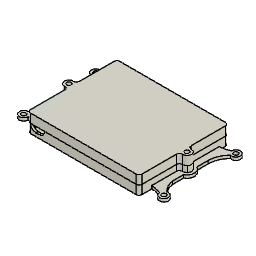
bat case v9 (Autodesk Fusion 360 design; units mm, degrees)
Autodesk Fusion 360 part; units mm, degrees
note: some values were not read from the file. Chosen so that the rebuilt part matches the saved one: which bodies a step acts on; which face or edge a step refers to; which pieces of a blend or face edit are solid. Set by a fixed rule: which sketch regions a step uses.
sketch "Sketch1" plane through (0, 0, 0) normal (0, 0, 1) x (1, 0, 0)
  line L0 (0, 0) -> (93.2, 0) construction
  line L1 (93.2, 0) -> (93.2, -48.6) construction
  line L2 (93.2, -48.6) -> (0, -48.6) construction
  line L3 (0, -48.6) -> (0, 0) construction
  line L4 (0, 0) -> (93.2, 0) construction
  line L5 (93.2, 0) -> (93.2, -48.6) construction
  line L6 (93.2, -48.6) -> (0, -48.6) construction
  line L7 (0, -48.6) -> (0, 0) construction
  line L8 (0, 0) -> (93.2, -48.6) construction
  line L9 (0, -48.6) -> (93.2, 0) construction
  line L10 (80.4585, 3.2151) -> (12.6326, -51.9036) construction
  line L11 (13.0397, 2.0949) -> (81.6326, -51.8528) construction
  circle A0 centre (93.2, 0) radius 1.5
  circle A1 centre (93.2, -48.6) radius 1.5
  circle A2 centre (0, -48.6) radius 1.5
  circle A3 centre (0, 0) radius 1.5
  circle A4 centre (0, 0) radius 3
  circle A5 centre (0, -48.6) radius 3
  circle A6 centre (93.2, -48.6) radius 3
  circle A7 centre (93.2, 0) radius 3
  line L12 (1.5, -2.5981) -> (1.5, -2.5138)
  line L13 (83.45, -54.15) -> (83.45, 3.05)
  line L14 (83.45, 3.05) -> (11.25, 3.05)
  line L15 (11.25, 3.05) -> (11.25, -54.15)
  line L16 (11.25, -54.15) -> (83.45, -54.15)
  line L17 (89.3079, -13.4947) -> (89.3079, -34.9816)
  line L18 (5.2688, -37.4913) -> (5.2688, -13.498)
  line L19 (9.7699, -1.523) -> (11.25, -1.523)
  line L20 (83.45, -1.523) -> (83.449, -1.523)
  line L21 (88.614, -49.274) -> (83.45, -49.274)
  line L22 (11.25, -47.288) -> (9.4012, -47.2941)
  arc A8 (9.4012, -47.2941) -> (2.9961, -48.7539) centre (9.4508, -62.2941) ccw
  arc A9 (5.2688, -13.498) -> (0.8586, -2.8745) centre (-9.7312, -13.498) ccw
  arc A10 (2.9986, 0.0924) -> (9.7699, -1.523) centre (9.7699, 13.477) ccw
  arc A11 (83.449, -1.523) -> (90.2011, 0.0827) centre (83.449, 13.477) ccw
  arc A12 (89.3079, -34.9816) -> (93.7677, -45.6542) centre (104.3079, -34.9816) ccw
  arc A13 (90.3003, -49.3691) -> (88.614, -49.274) centre (88.614, -64.274) ccw
  arc A14 (0.8858, -45.7338) -> (5.2688, -37.4913) centre (-8.9578, -35.2127) ccw
  arc A15 (92.3454, -2.8757) -> (89.3079, -13.4947) centre (104.6143, -12.1291) ccw
  line L23 (9.65, 4.65) -> (9.65, -55.75)
  line L24 (9.65, -55.75) -> (85.05, -55.75)
  line L25 (85.05, -55.75) -> (85.05, 4.65)
  line L26 (85.05, 4.65) -> (9.65, 4.65)
  point P0 (46.6, -24.3)
  dimension "d1" = 93.2
  dimension "d2" = 48.6
  dimension "d3" = 69
  dimension "d4" = 54
  dimension "d5" = 3
  dimension "d6" = 3
  dimension "d7" = 3
  dimension "d8" = 3
  dimension "d9" = 6
  dimension "d10" = 6
  dimension "d11" = 6
  dimension "d12" = 6
  dimension "d19" = 15
  dimension "d20" = 15
  dimension "d21" = 15
  dimension "d22" = 15
  dimension "d24" = 15
  dimension "d25" = 15
  dimension "d33" = 1.6
  constraint coincident L0.start L3.end
  constraint horizontal L0
  constraint perpendicular L0 L1
  constraint perpendicular L1 L2
  constraint perpendicular L0 L3
  constraint horizontal L4
  constraint vertical L5
  constraint horizontal L6
  constraint vertical L7
  constraint coincident L10 P0
  constraint coincident L11 P0
  constraint midpoint L9 P0
  constraint coincident L0.end L1.start
  constraint coincident L1.end L2.start
  constraint coincident L2.end L3.start
  constraint concentric A2 A5
  constraint concentric A1 A6
  constraint coincident A4 L12.start
  constraint vertical L17
  constraint perpendicular L15 L21
  constraint vertical L18
  constraint perpendicular L18 L19
  constraint collinear L19 L20
  constraint coincident L15 L19.end
  constraint coincident L13 L20.start
  constraint coincident L13 L21.end
  constraint coincident L15 L22.start
  constraint tangent L22 A8
  constraint tangent L18 A9
  constraint tangent L19 A10
  constraint tangent L20 A11
  constraint tangent L17 A12
  constraint tangent L21 A13
  constraint coincident A5 A14.start
  constraint coincident A5 A8.end
  constraint coincident A6 A13.start
  constraint coincident A6 A12.end
  constraint coincident A7 A15.start
  constraint coincident A7 A11.end
  constraint coincident A4 A10.start
  constraint coincident A4 A9.end
  measures "d1" distance of L0.start L0.end
  measures "d2" distance of L0.end L1.end
  measures "d3" distance of L10.end L11.end
  measures "d4" distance of L11.start L10.end
  measures "d5" diameter of A0
  measures "d6" diameter of A1
  measures "d7" diameter of A2
  measures "d8" diameter of A3
  measures "d9" diameter of A4
  measures "d10" diameter of A5
  measures "d11" diameter of A6
  measures "d12" diameter of A7
  measures "d19" radius of A8
  measures "d20" radius of A9
  measures "d21" radius of A10
  measures "d22" radius of A11
  measures "d24" radius of A12
  measures "d25" radius of A13
extrude "Extrude1" add sketch "Sketch1" along normal blind 2 contours A4 | A4 A5 L18 L22 A8 A9 A10 A14 L23 | L15 L19 L22 A10 L23 | L13 L14 L15 L16 | A5 | L13 L21 A11 L25 | A6 A7 L17 L21 A11 A12 A13 A15 L25 | A7 | A6 makes body 1
ref_plane "WorkPlane1" through (46.6003, -25.3245, 2) normal (0, 0, 1) x (1, 0, 0)
sketch "Sketch2" plane through (47.35, -25.55, 2) normal (0, 0, 1) x (1, 0, 0)
  line L0 (-36.1, -28.6) -> (36.1, -28.6)
  line L1 (36.1, -28.6) -> (36.1, 28.6)
  line L2 (-36.1, 28.6) -> (-36.1, -28.6)
  line L3 (36.1, 28.6) -> (-36.1, 28.6)
  line L4 (-37.7, 30.2) -> (-37.7, -30.2)
  line L5 (-37.7, -30.2) -> (37.7, -30.2)
  line L6 (37.7, -30.2) -> (37.7, 30.2)
  line L7 (37.7, 30.2) -> (-37.7, 30.2)
extrude "Extrude3" add sketch "Sketch2" along normal blind 10 separate body makes body 2
extrude "Extrude4" add sketch "Sketch2" against normal up to surface (2 mm away) bodies 1 2
fillet "Fillet2" radius 2 4 edges at (85.05, -55.75, 6) (9.65, -55.75, 6) (9.65, 4.65, 6) (85.05, 4.65, 6) on bodies 1
extrude "Extrude5" add 1 faces at (35.3167, -35.0833, 2) along direction (0, 0, 1) up to surface (10 mm away) on bodies 1 bodies 1
ref_plane "WorkPlane2" through (47.35, -25.55, 6) normal (0, 0, 1) x (1, 0, 0)
ref_plane "WorkPlane3" through (85.05, -25.55, 6) normal (1, 0, 0) x (0, 1, 0)
split "Split1" by plane through (85.05, -25.55, 6) normal (1, 0, 0) bodies 1 makes body 3 at (86.4693, -21.402, 0)
ref_plane "WorkPlane4" through (9.65, -25.55, 6) normal (-1, 0, 0) x (0, -1, 0)
split "Split2" by plane through (9.65, -25.55, 6) normal (-1, 0, 0) bodies 1 makes body 4 at (8.1896, -20.7713, 2)
shell "Shell1" thickness 1.6 removed faces 0 bodies 1
split "Split3" by plane through (47.35, -25.55, 6) normal (0, 0, 1) bodies 1 makes body 5 at (59.25, -35.6167, 12)
sketch "Sketch4" plane through (0, 0, 2) normal (0, 0, 1) x (-1, 0, 0)
  line L0 (-9.65, 47.2933) -> (-9.65, 1.5225)
  arc A0 (-2.9986, -0.0924) -> (-9.65, 1.5225) centre (-9.7699, -13.477) ccw
  arc A1 (-2.9986, -0.0924) -> (-0.8586, 2.8745) centre (0, 0) ccw
  arc A2 (-5.2688, 13.498) -> (-0.8586, 2.8745) centre (9.7312, 13.498) ccw
  line L1 (-5.2688, 13.498) -> (-5.2688, 37.4913)
  arc A3 (-0.8858, 45.7338) -> (-5.2688, 37.4913) centre (8.9578, 35.2127) ccw
  arc A4 (-0.8858, 45.7338) -> (-2.9961, 48.7539) centre (0, 48.6) ccw
  arc A5 (-9.4012, 47.2941) -> (-2.9961, 48.7539) centre (-9.4508, 62.2941) ccw
  circle A6 centre (0, 48.6) radius 1.5
  circle A7 centre (0, 0) radius 1.5
  arc A8 (-9.65, 21.0554) -> (-9.65, 30.0446) centre (-7.4594, 25.55) ccw
  circle A9 centre (-7.4594, 25.55) radius 1.5
  arc A10 (-9.65, 23.5003) -> (-9.65, 27.5997) centre (-7.4594, 25.55) ccw
  line L2 (-9.4012, 47.2941) -> (-9.65, 47.2933)
  dimension "d51" = 10
  dimension "d52" = 6
  dimension "d53" = 3
  constraint coincident L0 A8.end
  constraint coincident L0 A8.start
  constraint concentric A8 A10
  constraint concentric A8 A9
  constraint coincident L0 A10.end
  constraint coincident L0 A10.start
  measures "d51" diameter of A8
  measures "d52" diameter of A10
  measures "d53" diameter of A9
extrude "Extrude7" add sketch "Sketch4" against normal blind 2 contours L1 A8 A10 | L1 A10 bodies 4
extrude "Extrude8" add sketch "Sketch4" along normal blind 4 contours L0 L1 A10 | L1 A10 bodies 1 4 5
extrude "Extrude9" add 1 faces at (9.4198, -25.55, 6) along direction (0, 0, 1) blind 6 on bodies 1 bodies 1
ref_plane "WorkPlane5" through (9.65, -25.55, 6) normal (-1, 0, 0) x (0, -1, 0)
split "Split4" by plane through (9.65, -25.55, 6) normal (-1, 0, 0) bodies 1 makes body 6 at (8.1896, -23.2904, 0)
ref_plane "WorkPlane6" through (47.35, -25.55, 6) normal (-1, 0, 0) x (0, -1, 0)
mirror "Mirror1" about plane through (47.35, -25.55, 6) normal (-1, 0, 0) of bodies 6 makes body 7
combine "Combine1" operation add target body 3 tool bodies 1 6 7
ref_plane "WorkPlane7" through (47.35, -25.55, 6) normal (0, 0, 1) x (1, 0, 0)
split "Split5" by plane through (47.35, -25.55, 6) normal (0, 0, 1) bodies 3 makes body 8 at (59.25, -14.1169, 12)
sketch "Sketch5" plane through (9.65, 0, 0) normal (-1, 0, 0) x (0, -1, 0)
  line L0 (27.5997, 6) -> (53.75, 6)
  line L1 (53.75, 6) -> (53.75, 12)
  line L2 (53.75, 12) -> (27.5997, 12)
  line L3 (27.5997, 12) -> (27.5997, 6)
sketch "Sketch6" plane through (0, -55.75, 0) normal (0, -1, 0) x (1, 0, 0)
  line L0 (11.65, 6) -> (83.05, 6)
  line L1 (83.05, 6) -> (83.05, 12)
  line L2 (83.05, 12) -> (11.65, 12)
  line L3 (11.65, 12) -> (11.65, 6)
  line L4 (17.5813, 9.7242) -> (15.3644, 9.7242)
  arc A0 (15.3644, 9.7242) -> (15.3644, 2.2758) centre (15.3644, 6) ccw
  line L5 (15.3644, 2.2758) -> (17.5813, 2.2758)
  arc A1 (17.5813, 2.2758) -> (17.5813, 9.7242) centre (17.5813, 6) ccw
  line L6 (17.5813, 6) -> (15.3644, 6) construction
  constraint tangent L4 A0
  constraint tangent A0 L5
  constraint parallel L4 L5
  constraint tangent L5 A1
  constraint tangent L4 A1
  constraint coincident L0 A0.centre
  constraint perpendicular L3 L6
extrude "Extrude10" cut sketch "Sketch6" against normal up to surface (1.6 mm away) contours L0 L3 A0 L5 A1 bodies 3
fillet "Fillet3" radius 2 5 edges at (9.65, -27.5997, 4) (4.4594, -25.55, 2) (9.65, -23.5003, 4) (9.65, -27.5997, 9) (9.65, -23.5003, 9) on bodies 3 8
fillet "Fillet4" radius 2 5 edges at (90.2406, -25.55, 2) (85.05, -27.5997, 4) (85.05, -23.5003, 4) (85.05, -27.5997, 9) (85.05, -23.5003, 9) on bodies 3 8
delete_face "DeleteFace3" 1 faces at (6.9714, -20.9419, 2.0337) on bodies 3
delete_face "DeleteFace4" 1 faces at (89.0602, -29.8117, 2.0337) on bodies 3
move_body "Move1" bodies 8 to x (1, 0, 0) y (0, 1, 0) z (0, 0, 1) at (100, 0, 0)
move_body "Move2" bodies 8 to x (1, 0, 0) y (0, -1, 0) z (0, 0, -1) at (0, -51.1, 24)
move_body "Move3" bodies 8 to x (-1, 0, 0) y (0, 1, 0) z (0, 0, -1) at (198.9188, 0, 24)
move_body "Move4" bodies 8 to x (1, 0, 0) y (0, 1, 0) z (0, 0, 1) at (-4.2188, 0, -6)
move_body "Move5" bodies 8 to x (1, 0, 0) y (0, 1, 0) z (0, 0, 1) at (0, 0, 6)
delete_face "DeleteFace5" 1 faces at (86.5526, -11.1813, 2) on bodies 3
ref_plane "WorkPlane8" through (9.65, -40.6749, 9) normal (-1, 0, 0) x (0, -1, 0)
split "Split6" by plane through (9.65, -40.6749, 9) normal (-1, 0, 0) bodies 3 makes body 9 at (8.1896, -23.2904, 0)
mirror "Mirror2" about plane through (47.35, -25.55, 6) normal (-1, 0, 0) of bodies 9 makes body 10
named bodies: "bot", "top", "bot (1)", "bot (1) (1)"
